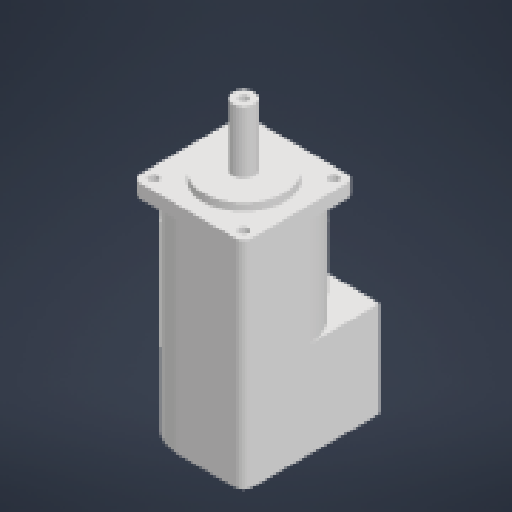
# Autodesk Inventor part: ServoMotor
Saved by Autodesk Inventor 2026 (Build 300175050, 175E)
## iProperties
Created: 2026-04-30
Part Number: ServoMotor
Material: Generic
Document SubType Name: Modeling
Designer: sniel
Density: 1 g/cm^3
Appearance: Default
Author: sniel
Autodesk Inventor part; units mm, degrees
ref_plane "YZ Plane" through (0, 0, 0) normal (1, 0, 0) x (0, 1, 0)
ref_plane "XZ Plane" through (0, 0, 0) normal (0, 1, 0) x (-1, 0, 0)
ref_plane "XY Plane" through (0, 0, 0) normal (0, 0, 1) x (1, 0, 0)
sketch "Sketch1" plane through (0, 0, 0) normal (0, 1, 0) x (-1, 0, 0)
  line L0 (-20.425, 20.425) -> (20.425, 20.425)
  line L1 (20.425, 20.425) -> (20.425, -20.425)
  line L2 (20.425, -20.425) -> (-20.425, -20.425)
  line L3 (-20.425, -20.425) -> (-20.425, 20.425)
  line L4 (-20.425, 20.425) -> (20.425, -20.425) construction
  line L5 (20.425, 20.425) -> (-20.425, -20.425) construction
  point P0 (0, 0)
  dimension "d0" = 40.85
  dimension "d1" = 40.85
  constraints: 12 end point, 2 midpoint, 2 parallel, 1 horizontal, 1 perpendicular
  measures "d0" distance of L1.end L2.end
  measures "d1" distance of L0.end L1.end
extrude "Extrusion1" add sketch "Sketch1" along normal blind 5
sketch "Sketch2" plane through (0, 5, 0) normal (0, 1, 0) x (1, 0, 0)
  line L0 (-20.425, 20.425) -> (-20.425, -20.425) projected
  line L1 (-20.425, -20.425) -> (-16.425, -20.425)
  line L2 (-16.425, -20.425) -> (-16.425, -16.425)
  line L3 (-16.425, -16.425) -> (-20.425, -16.425)
  line L4 (-20.425, -16.425) -> (-20.425, -20.425)
  line L5 (-20.425, 20.425) -> (-16.425, 20.425)
  line L6 (-16.425, 20.425) -> (-16.425, 16.425)
  line L7 (-16.425, 16.425) -> (-20.425, 16.425)
  line L8 (-20.425, 16.425) -> (-20.425, 20.425)
  line L9 (-20.425, -20.425) -> (20.425, -20.425) projected
  line L10 (20.425, -20.425) -> (16.425, -20.425)
  line L11 (16.425, -20.425) -> (16.425, -16.425)
  line L12 (16.425, -16.425) -> (20.425, -16.425)
  line L13 (20.425, -16.425) -> (20.425, -20.425)
  line L14 (20.425, 20.425) -> (16.425, 20.425)
  line L15 (16.425, 20.425) -> (16.425, 16.425)
  line L16 (16.425, 16.425) -> (20.425, 16.425)
  line L17 (20.425, 16.425) -> (20.425, 20.425)
  circle A0 centre (-16.425, -16.425) radius 1.75
  circle A1 centre (-16.425, 16.425) radius 1.75
  circle A2 centre (16.425, -16.425) radius 1.75
  circle A3 centre (16.425, 16.425) radius 1.75
  point P0 (0, 0)
  dimension "d4" = 4
  dimension "d5" = 4
  dimension "d6" = 4
  dimension "d7" = 4
  dimension "d8" = 4
  dimension "d9" = 4
  dimension "d10" = 4
  dimension "d11" = 4
  dimension "d12" = 3.5
  dimension "d13" = 3.5
  dimension "d14" = 3.5
  dimension "d15" = 3.5
  constraints: 32 end point, 8 parallel, 4 centre point, 4 coincident, 4 horizontal, 4 perpendicular, 2 point on line
  measures "d4" distance of L3.end L2.end
  measures "d5" distance of L2.end L1.end
  measures "d6" distance of L6.end L7.end
  measures "d7" distance of L5.end L6.end
  measures "d8" distance of L11.end L12.end
  measures "d9" distance of L10.end L11.end
  measures "d10" distance of L16.end L15.end
  measures "d11" distance of L15.end L14.end
  measures "d12" diameter of A0
  measures "d13" diameter of A1
  measures "d14" diameter of A2
  measures "d15" diameter of A3
extrude "Extrusion2" cut sketch "Sketch2" against normal blind 5 contours A1 L6 L7 | L7 L6 A1 | A0 L2 L3 | L3 L2 A0 | A2 L12 L11 | L11 L12 A2 | A3 L16 L15 | L15 L16 A3
fillet "Fillet1" radius 3 4 edges at (-20.425, 2.5, 20.425) (20.425, 2.5, 20.425) (20.425, 2.5, -20.425) (-20.425, 2.5, -20.425)
sketch "Sketch3" plane through (0, 5, 0) normal (0, 1, 0) x (1, 0, 0)
  circle A0 centre (0, 0) radius 14.875
  dimension "d19" = 29.75
  constraints: 1 centre point, 1 coincident
  measures "d19" diameter of A0
extrude "Extrusion3" add sketch "Sketch3" along normal blind 2.8
sketch "Sketch4" plane through (0, 7.8, 0) normal (0, 1, 0) x (1, 0, 0)
  circle A0 centre (0, 0) radius 3.925
  dimension "d22" = 7.85
  constraints: 1 centre point, 1 coincident
  measures "d22" diameter of A0
extrude "Extrusion4" add sketch "Sketch4" along normal blind 22.65
sketch "Sketch5" plane through (0, 30.45, 0) normal (0, 1, 0) x (1, 0, 0)
  circle A0 centre (0, 0) radius 3.925 projected
  circle A1 centre (0, 0) radius 1.5
  dimension "d25" = 3
  constraints: 1 centre point, 1 coincident
  measures "d25" diameter of A1
extrude "Extrusion5" cut sketch "Sketch5" against normal blind 22.65 contours A1
sketch "Sketch6" plane through (0, 0, 0) normal (0, -1, 0) x (1, 0, 0)
  arc A0 (-20.425, -17.425) -> (-17.425, -20.425) centre (-17.425, -17.425) ccw
  line L0 (17.425, -20.425) -> (-17.425, -20.425)
  arc A1 (17.425, -20.425) -> (20.425, -17.425) centre (17.425, -17.425) ccw
  line L1 (20.425, 17.425) -> (20.425, -17.425)
  arc A2 (20.425, 17.425) -> (17.425, 20.425) centre (17.425, 17.425) ccw
  line L2 (-17.425, 20.425) -> (17.425, 20.425)
  arc A3 (-17.425, 20.425) -> (-20.425, 17.425) centre (-17.425, 17.425) ccw
  line L3 (-20.425, -17.425) -> (-20.425, 17.425)
  line L4 (17.425, -20.425) -> (20.425, -20.425)
  arc A4 (17.425, -20.425) -> (20.425, -17.425) centre (17.425, -17.425) ccw
  line L5 (20.425, -20.425) -> (20.425, -17.425)
  circle A5 centre (16.425, -16.425) radius 1.75
  line L6 (16.425, -16.425) -> (0, 0)
  line L7 (16.425, -16.425) -> (15.3643, -15.3643)
  line L8 (20.425, 0) -> (20.425, -2.5)
  line L9 (20.425, 17.425) -> (20.425, -17.425)
  line L10 (0, -20.425) -> (2.5, -20.425)
  arc A6 (2.5, -20.425) -> (20.425, -2.5) centre (3.12, -3.12) ccw
  arc A7 (-2.5, 20.425) -> (-20.425, 2.5) centre (-3.12, 3.12) ccw
  point P0 (3.74, -20.425)
  point P1 (20.425, -3.74)
  point P2 (-3.74, 20.425)
  point P3 (-20.425, 3.74)
  dimension "d30" = 1.5
  dimension "d31" = 2.5
  dimension "d32" = 2.5
  constraints: 22 end point, 15 point on circle, 12 centre point, 3 point on line, 2 midpoint
  measures "d30" distance of L6.start L7.end
  measures "d31" distance of L8.start L8.end
  measures "d32" distance of L10.start L10.end
extrude "Extrusion6" add sketch "Sketch6" along normal blind 74 contours L3 A7 L2 A2 L1 A6 A5 L0 A0 | A5 L6 A6 | A5 A6 L6
sketch "Sketch7" plane through (0, -74, 0) normal (0, -1, 0) x (1, 0, 0)
  line L0 (-17.425, -20.425) -> (3.74, -20.425)
  arc A0 (3.74, -20.425) -> (20.425, -3.74) centre (3.12, -3.12) ccw
  line L1 (20.425, -3.74) -> (20.425, 17.425)
  arc A1 (20.425, 17.425) -> (17.425, 20.425) centre (17.425, 17.425) ccw
  line L2 (17.425, 20.425) -> (-3.74, 20.425)
  arc A2 (-3.74, 20.425) -> (-20.425, 3.74) centre (-3.12, 3.12) ccw
  line L3 (-20.425, 3.74) -> (-20.425, -17.425)
  arc A3 (-20.425, -17.425) -> (-17.425, -20.425) centre (-17.425, -17.425) ccw
  arc A4 (3.74, -20.425) -> (20.425, -3.74) centre (3.12, -3.12) ccw projected
  line L4 (20.425, -3.74) -> (20.425, -20.425)
  line L5 (-17.425, -20.425) -> (3.74, -20.425) projected
  line L6 (20.425, -20.425) -> (3.74, -20.425)
  line L7 (20.425, -20.425) -> (20.425, -29.425)
  line L8 (20.425, -29.425) -> (-20.425, -29.425)
  line L9 (-20.425, -29.425) -> (-20.425, -17.425)
  point P0 (0, 0)
  dimension "d33" = 9
  constraints: 18 end point, 8 centre point, 8 point on circle, 2 perpendicular, 2 vertical, 1 collinear
  measures "d33" distance of L4.end L7.end
extrude "Extrusion7" add sketch "Sketch7" against normal blind 35
sketch "Sketch8" plane through (0, 5, 0) normal (0, 1, 0) x (1, 0, 0)
  circle A0 centre (-16.425, -16.425) radius 1.75 projected
  circle A1 centre (-16.425, 16.425) radius 1.75 projected
  circle A2 centre (16.425, -16.425) radius 1.75 projected
  circle A3 centre (16.425, 16.425) radius 1.75 projected
  point P0 (0, 0)
extrude "Extrusion8" cut sketch "Sketch8" against normal blind 13 contours A0 | A3
body "Solid1"
